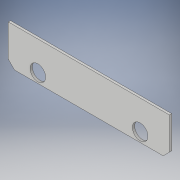
# Autodesk Inventor part: MecanumDriveTrainPlate17-18
Saved by Autodesk Inventor 2017 (Build 210142000, 142)
## iProperties
Created: 2017-09-16
Part Number: MecanumDriveTrainPlate17-18
Material: Generic
Document SubType Name: Modeling
Designer: User
Density: 1 g/cm^3
Appearance: Default
Author: User
Autodesk Inventor part; units mm, degrees
ref_plane "YZ Plane" through (0, 0, 0) normal (1, 0, 0) x (0, 1, 0)
ref_plane "XZ Plane" through (0, 0, 0) normal (0, 1, 0) x (-1, 0, 0)
ref_plane "XY Plane" through (0, 0, 0) normal (0, 0, 1) x (1, 0, 0)
sketch "Sketch1" plane through (0, 0, 0) normal (0, 0, 1) x (1, 0, 0)
  line L0 (0, 0) -> (444.5, 0)
  line L1 (444.5, 0) -> (444.5, 127)
  line L2 (444.5, 127) -> (0, 127)
  line L3 (0, 127) -> (0, 0)
  dimension "d0" = 444.5
  dimension "d1" = 127
  constraints: 8 end point, 2 perpendicular, 1 horizontal, 1 vertical
  measures "d0" distance of L0.start L0.end
  measures "d1" distance of L0.end L1.end
extrude "Extrusion1" add sketch "Sketch1" along normal blind 6.35
sketch "Sketch2" plane through (0, 0, 6.35) normal (0, 0, 1) x (1, 0, 0)
  line L0 (0, 0) -> (444.5, 0) projected
  line L1 (38.0923, 0) -> (0, 38.0919)
  line L2 (0, 127) -> (0, 0) projected
  line L3 (0, 0) -> (444.5, 0) projected
  line L4 (444.5, 0) -> (444.5, 127) projected
  line L5 (444.5, 0) -> (406.4, 0)
  line L6 (444.5, 0) -> (482.6, 0) construction
  line L7 (444.5, 0) -> (444.5, 38.0919)
  line L8 (444.5, 38.0919) -> (406.4086, 0)
  point P0 (419.1126, 0)
  dimension "d19" = 38.1
  dimension "d20" = 180
  constraints: 10 end point, 5 point on line, 3 collinear, 1 horizontal
  measures "d19" distance of L0.end L5.end
  measures "d20" angle of L5 L6
extrude "Extrusion2" cut sketch "Sketch2" against normal blind 50.8
sketch "Sketch3" plane through (0, 0, 6.35) normal (0, 0, 1) x (1, 0, 0)
  line L0 (0, 77.664) -> (80.645, 77.664) construction
  line L1 (444.5, 127) -> (0, 127) projected
  line L2 (80.645, 127) -> (161.29, 127) construction
  circle A0 centre (81.534, 46.355) radius 21.59
  line L3 (444.5, 38.0919) -> (444.5, 127) projected
  line L4 (444.5, 77.664) -> (525.145, 77.664) construction
  line L5 (444.5, 38.0919) -> (444.5, 127) projected
  line L6 (444.5, 46.355) -> (525.145, 46.355) construction
  circle A1 centre (363.855, 46.355) radius 21.59
  line L7 (444.5, 127) -> (0, 127) projected
  line L8 (0, 127) -> (0, 38.0919) projected
  circle A2 centre (58.2577, 38.8774) radius 1.8542
  circle A3 centre (58.3621, 41.6798) radius 1.8288
  circle A4 centre (104.5311, 39.3446) radius 1.8542
  circle A5 centre (104.7028, 53.3654) radius 1.8542
  point P0 (0, 0)
  dimension "d10" = 43.18
  dimension "d18" = 43.18
  dimension "d40" = 46.228
  dimension "d41" = 3.7084
  dimension "d42" = 3.6576
  dimension "d43" = 3.7084
  dimension "d44" = 3.7084
  dimension "d45" = 80.645
  dimension "d46" = 80.645
  dimension "d47" = 73.6346
  dimension "d48" = 14.0208
  dimension "d49" = 2.8024
  constraints: 8 end point, 6 centre point, 4 coincident, 4 horizontal, 3 point on line
  measures "d10" diameter of A0
  measures "d18" diameter of A1
  measures "d40" distance of point (58.362, 41.68) point (104.531, 39.345)
  measures "d41" diameter of A2
  measures "d42" diameter of A3
  measures "d43" diameter of A4
  measures "d44" diameter of A5
  measures "d45" distance from line of L1 A0.centre
  measures "d46" distance from line of L1 A1.centre
  measures "d47" distance from line of L1 A5.centre
  measures "d48" vertical distance of A4.centre A5.centre
  measures "d49" vertical distance of A3.centre A2.centre
extrude "Extrusion3" cut sketch "Sketch3" against normal blind 50.8 contours A0 | A1
thicken "Thicken1" operation add thickness 20.828 both sides no extend neighbours yes toward (0, 1, 0) faces at (160.8644, 0, 2.1167)
body "Solid1"
